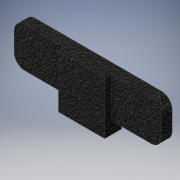
# Autodesk Inventor part: RotationLock
Saved by Autodesk Inventor 2019 (Build 230136000, 136)
## iProperties
Created: 2019-05-08
Part Number: RotationLock
Material: Generic
Document SubType Name: Modeling
Designer: Iván
Density: 1 g/cm^3
Appearance: Default
Mass: 8.60137 g
Surface Area: 42.2096 cm^2
Volume: 8.60137 cm^3
Author: Iván
Autodesk Inventor part; units mm, degrees
ref_plane "YZ Plane" through (0, 0, 0) normal (1, 0, 0) x (0, 1, 0)
ref_plane "XZ Plane" through (0, 0, 0) normal (0, 1, 0) x (-1, 0, 0)
ref_plane "XY Plane" through (0, 0, 0) normal (0, 0, 1) x (1, 0, 0)
sketch "Sketch1" plane through (0, 0, 0) normal (0, 0, 1) x (1, 0, 0)
  line L0 (-350, 95) -> (350, 95)
  line L1 (350, 95) -> (350, -95)
  line L2 (350, -95) -> (-350, -95)
  line L3 (-350, -95) -> (-350, 95)
  circle A0 centre (-250, 55) radius 10
  circle A1 centre (-250, -15) radius 10
  circle A2 centre (250, 55) radius 10
  circle A3 centre (250, -15) radius 10
  line L4 (-110, 95) -> (110, 95)
  point P0 (0, 0)
  point P1 (0, 95)
  point P2 (350, 0)
  point P3 (0, -155)
  dimension "d0" = 700
  dimension "d1" = 190
  dimension "d2" = 20
  dimension "d3" = 70
  dimension "d4" = 40
  dimension "d7" = 20
  dimension "d8" = 70
  dimension "d9" = 500
  dimension "d10" = 100
  constraints: 10 end point, 4 centre point, 4 vertical alignment, 2 equal radius, 2 horizontal, 2 horizontal alignment, 2 midpoint, 2 parallel, 1 collinear, 1 perpendicular
  measures "d0" distance of L0.start L0.end
  measures "d1" distance of L0.end L1.end
  measures "d2" diameter of A0
  measures "d3" distance of A1.centre A0.centre
  measures "d4" distance from line of L0 A0.centre
  measures "d7" diameter of A2
  measures "d8" distance of A3.centre A2.centre
  measures "d9" distance of A2.centre A0.centre
  measures "d10" distance from line of L3 A0.centre
extrude "Extrusion1" add sketch "Sketch1" along normal blind 50
sketch "Sketch2" plane through (0, 0, 50) normal (0, 0, 1) x (1, 0, 0)
  line L0 (-110, 95) -> (110, 95)
  line L1 (110, 95) -> (110, -155)
  line L2 (110, -155) -> (-110, -155)
  line L3 (-110, -155) -> (-110, 95)
  line L4 (350, 95) -> (-350, 95) projected
  point P0 (0, 0)
  point P1 (0, -155)
  dimension "d15" = 220
  dimension "d16" = 250
  constraints: 8 end point, 2 parallel, 1 collinear, 1 horizontal, 1 midpoint, 1 perpendicular, 1 vertical alignment
  measures "d15" distance of L0.start L0.end
  measures "d16" distance of L0.end L1.end
extrude "Extrusion2" add sketch "Sketch2" along normal blind 30
sketch "Sketch3" plane through (0, 0, 50) normal (0, 0, -1) x (-1, 0, 0)
  line L0 (110, -95) -> (-110, -95) projected
  line L1 (-110, -95) -> (-110, -155) projected
  line L2 (-110, -155) -> (110, -155) projected
  line L3 (110, -155) -> (110, -95) projected
  point P0 (0, 0)
extrude "Extrusion3" add sketch "Sketch3" along normal blind 50
fillet "Fillet1" radius 50 4 edges at (-350, -95, 25) (-350, 95, 25) (350, -95, 25) (350, 95, 25)
scale "Scale1" factors (0.1, 0.1, 0.1) then translate (-225, -13.5, 0) bodies 1
equation "\"d7\" = d2"
equation "\"d10\" = -0.5 * d9 + 0.5 * d0"
body "Solid1"
